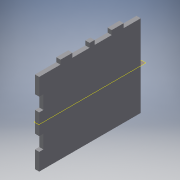
# Autodesk Inventor part: Part9
Saved by Autodesk Inventor 2018 (Build 220112000, 112)
## iProperties
Created: 2018-05-22
Part Number: Part9
Material: Generic
Document SubType Name: Modeling
Designer: Administrator
Density: 1 g/cm^3
Appearance: Default
Author: Administrator
Autodesk Inventor part; units mm, degrees
ref_plane "YZ Plane" through (0, 0, 0) normal (1, 0, 0) x (0, 1, 0)
ref_plane "XZ Plane" through (0, 0, 0) normal (0, 1, 0) x (-1, 0, 0)
ref_plane "XY Plane" through (0, 0, 0) normal (0, 0, 1) x (1, 0, 0)
sketch "Sketch1" plane through (0, 0, 0) normal (1, 0, 0) x (0, 1, 0)
  line L0 (33.2271, 21.6336) -> (-27.7329, 21.6336)
  line L1 (-27.7329, 21.6336) -> (-27.7329, -50.7564)
  line L2 (-27.7329, -50.7564) -> (33.2271, -50.7564)
  line L3 (33.2271, -50.7564) -> (33.2271, 21.6336)
  line L4 (33.2271, -38.0564) -> (36.4021, -38.0564)
  line L5 (36.4021, -38.0564) -> (36.4021, -29.1664)
  line L6 (36.4021, -29.1664) -> (33.2271, -29.1664)
  line L7 (33.2271, -29.1664) -> (33.2271, -38.0564)
  line L8 (33.2271, 8.9336) -> (36.4021, 8.9336)
  line L9 (36.4021, 8.9336) -> (36.4021, 0.0436)
  line L10 (36.4021, 0.0436) -> (33.2271, 0.0436)
  line L11 (33.2271, 0.0436) -> (33.2271, 8.9336)
  line L12 (33.2271, -16.4664) -> (36.4021, -16.4664)
  line L13 (36.4021, -16.4664) -> (36.4021, -12.6564)
  line L14 (36.4021, -12.6564) -> (33.2271, -12.6564)
  line L15 (33.2271, -12.6564) -> (33.2271, -16.4664)
  line L16 (33.2271, 21.6336) -> (20.5271, 21.6336)
  line L17 (20.5271, 21.6336) -> (20.5271, 24.8086)
  line L18 (20.5271, 24.8086) -> (33.2271, 24.8086)
  line L19 (33.2271, 24.8086) -> (33.2271, 21.6336)
  line L20 (-27.7329, 21.6336) -> (-15.0329, 21.6336)
  line L21 (-15.0329, 21.6336) -> (-15.0329, 24.8086)
  line L22 (-15.0329, 24.8086) -> (-27.7329, 24.8086)
  line L23 (-27.7329, 24.8086) -> (-27.7329, 21.6336)
  line L24 (-4.8729, 21.6336) -> (10.3671, 21.6336)
  line L25 (10.3671, 21.6336) -> (10.3671, 24.8086)
  line L26 (10.3671, 24.8086) -> (-4.8729, 24.8086)
  line L27 (-4.8729, 24.8086) -> (-4.8729, 21.6336)
  point P0 (0, 0)
  dimension "d0" = 60.96
  dimension "d1" = 72.39
  dimension "d2" = 12.7
  dimension "d3" = 8.89
  dimension "d4" = 3.175
  dimension "d5" = 8.89
  dimension "d6" = 12.7
  dimension "d7" = 12.7
  dimension "d8" = 12.7
  dimension "d11" = 3.175
  dimension "d12" = 12.7
  dimension "d13" = 12.7
  dimension "d14" = 10.16
  dimension "d15" = 10.16
  constraints: 56 end point, 14 parallel, 7 horizontal, 7 perpendicular, 4 point on line
  measures "d0" distance between parallel lines of L1 L3
  measures "d1" distance between parallel lines of L0 L2
  measures "d2" distance between parallel lines of L4 L2
  measures "d3" distance between parallel lines of L6 L4
  measures "d4" distance between parallel lines of L3 L5
  measures "d5" distance between parallel lines of L8 L10
  measures "d6" distance between parallel lines of L0 L8
  measures "d7" distance between parallel lines of L12 L6
  measures "d8" distance between parallel lines of L10 L14
  measures "d11" distance between parallel lines of L18 L16
  measures "d12" distance between parallel lines of L17 L19
  measures "d13" distance between parallel lines of L23 L21
  measures "d14" distance between parallel lines of L21 L27
  measures "d15" distance between parallel lines of L25 L17
ref_plane "Work Plane1" through (0, 2.7471, 0.0436) normal (0, 1, 0) x (1, 0, 0)
extrude "Extrusion3" add sketch "Sketch1" along normal blind 3.175
ref_plane "Work Plane2" through (0, -15.0329, -14.5614) normal (0, 0, 1) x (1, 0, 0)
mirror "Mirror2" about plane through (0, -15.0329, -14.5614) normal (0, 0, 1) of "Extrusion3"
mirror "Mirror3" about plane through (0, 2.7471, 0.0436) normal (0, 1, 0) of "Extrusion3"
body "Solid3"
